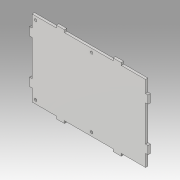
# Autodesk Inventor part: bottom_instrumentboard
Saved by Autodesk Inventor 2019.3 (Build 233278000, 278)
## iProperties
Created: 2019-05-28
Part Number: bottom_instrumentboard
Material: Generic
Document SubType Name: Modeling
Designer: Dave
Density: 1 g/cm^3
Appearance: Default
Author: Dave
Autodesk Inventor part; units mm, degrees
ref_plane "YZ Plane" through (0, 0, 0) normal (1, 0, 0) x (0, 1, 0)
ref_plane "XZ Plane" through (0, 0, 0) normal (0, 1, 0) x (-1, 0, 0)
ref_plane "XY Plane" through (0, 0, 0) normal (0, 0, 1) x (1, 0, 0)
sketch "Sketch1" plane through (0, 0, 0) normal (0, 0, 1) x (1, 0, 0)
  line L0 (0, 0) -> (140, 0)
  line L1 (140, 0) -> (140, 94)
  line L2 (140, 94) -> (0, 94)
  line L3 (0, 94) -> (0, 0)
  circle A0 centre (4.5, 89.5) radius 1.55
  circle A1 centre (4.5, 4.5) radius 1.55
  circle A2 centre (73.5, 89.5) radius 1.55
  circle A3 centre (73.5, 4.5) radius 1.55
  line L4 (0, 79) -> (-3, 79)
  line L5 (-3, 79) -> (-3, 69)
  line L6 (-3, 69) -> (0, 69)
  line L7 (0, 69) -> (0, 79)
  line L8 (0, 25) -> (-3, 25)
  line L9 (-3, 25) -> (-3, 15)
  line L10 (-3, 15) -> (0, 15)
  line L11 (0, 15) -> (0, 25)
  line L12 (140, 79) -> (143, 79)
  line L13 (143, 79) -> (143, 69)
  line L14 (143, 69) -> (140, 69)
  line L15 (140, 69) -> (140, 79)
  line L16 (140, 25) -> (143, 25)
  line L17 (143, 25) -> (143, 15)
  line L18 (143, 15) -> (140, 15)
  line L19 (140, 15) -> (140, 25)
  line L20 (30, 94) -> (40, 94)
  line L21 (40, 94) -> (40, 97)
  line L22 (40, 97) -> (30, 97)
  line L23 (30, 97) -> (30, 94)
  line L24 (100, 94) -> (110, 94)
  line L25 (110, 94) -> (110, 97)
  line L26 (110, 97) -> (100, 97)
  line L27 (100, 97) -> (100, 94)
  line L28 (30, 0) -> (40, 0)
  line L29 (40, 0) -> (40, -3)
  line L30 (40, -3) -> (30, -3)
  line L31 (30, -3) -> (30, 0)
  line L32 (100, 0) -> (110, 0)
  line L33 (110, 0) -> (110, -3)
  line L34 (110, -3) -> (100, -3)
  line L35 (100, -3) -> (100, 0)
  point P0 (141.5, 25)
  point P1 (-1.5, 25)
  point P2 (-1.5, 69)
  point P3 (141.5, 69)
  point P4 (-3, 74)
  point P5 (-3, 20)
  point P6 (143, 74)
  point P7 (143, 20)
  dimension "d0" = 3.1
  dimension "d1" = 85
  dimension "d2" = 69
  dimension "d3" = 94
  dimension "d4" = 4.5
  dimension "d5" = 4.5
  dimension "d6" = 4.5
  dimension "d7" = 140
  dimension "d8" = 3
  dimension "d9" = 10
  dimension "d10" = 15
  dimension "d11" = 15
  dimension "d12" = 30
  dimension "d13" = 30
  constraints: 72 end point, 19 point on line, 18 parallel, 9 horizontal, 9 perpendicular, 8 midpoint, 6 equal length, 4 centre point, 4 horizontal alignment, 4 vertical alignment, 3 equal radius, 1 collinear
  measures "d0" diameter of A0
  measures "d1" distance of A1.centre A0.centre
  measures "d2" distance of A2.centre A0.centre
  measures "d3" distance between parallel lines of L0 L2
  measures "d4" distance from line of L0 A1.centre
  measures "d5" distance from line of L2 A0.centre
  measures "d6" distance from line of L3 A0.centre
  measures "d7" distance between parallel lines of L1 L3
  measures "d8" distance of L4.start L4.end
  measures "d9" distance of L4.end L5.end
  measures "d10" distance between parallel lines of L2 L4
  measures "d11" distance between parallel lines of L0 L10
  measures "d12" distance between parallel lines of L3 L23
  measures "d13" distance between parallel lines of L1 L25
extrude "Extrusion1" add sketch "Sketch1" along normal blind 3
body "Solid1"
